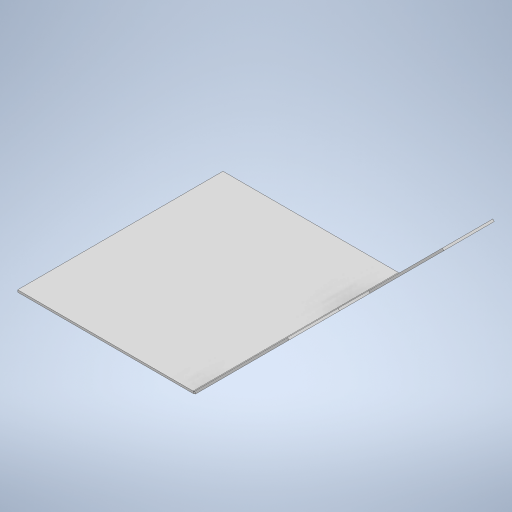
# Autodesk Inventor part: LzC-FrontPLateRS3
Saved by Autodesk Inventor 2024.3 (Build 283343000, 343)
## iProperties
Created: 2025-06-17
Part Number: LzC-FrontPLateRS3
Material: Generic
Document SubType Name: Sheet Metal
Designer: ajclo
Density: 1 g/cm^3
Sheet Metal Rule: Default_mm
Appearance: Default
Flat Pattern Width: 19.7 cm
Flat Pattern Length: 29.6736 cm
Flat Pattern Area: 584.57 cm^2
Sheet Metal Width: 197,000 mm
Sheet Metal Length: 296,736 mm
Sheet Metal Area: 58457,039 mm^2
Author: ajclo
Autodesk Inventor part; units mm, degrees
ref_plane "YZ Plane" through (0, 0, 0) normal (1, 0, 0) x (0, 1, 0)
ref_plane "XZ Plane" through (0, 0, 0) normal (0, 1, 0) x (-1, 0, 0)
ref_plane "XY Plane" through (0, 0, 0) normal (0, 0, 1) x (1, 0, 0)
sketch "Sketch1" plane through (0, 0, 0) normal (0, 1, 0) x (-1, 0, 0)
  line L0 (0, 0) -> (169.946, 0)
  line L1 (169.946, 0) -> (169.946, -197)
  line L2 (169.946, -197) -> (0, -197)
  line L3 (0, -197) -> (0, 0)
  dimension "d0" = 197
  dimension "d1" = 169.946
  measures "d0" distance of L0.end L1.end
  measures "d1" distance of L1.end L2.end
extrude "Plate1" add sketch "Sketch1" along normal blind 2
sketch "Sketch2" plane through (-1.4142, 1.4142, -197) normal (0.7071068, -0.7071068, 0) x (0.7071068, 0.7071068, 0)
  line L0 (0, 197) -> (0, 0)
  line L1 (0, 0) -> (127.842, 0)
  line L2 (127.842, 0) -> (127.842, 197)
  line L3 (127.842, 197) -> (0, 197)
  constraints: 6 end point, 1 horizontal, 1 perpendicular, 1 vertical
edge flange "Flange1" height 127.842 angle 45 thickness 2 bend radius 2 thickness toward (0.7071068, -0.7071068, 0) relief straight relief width 2 relief depth 1 edges at (0, 2, -98.5) wall of the first edge with corners at (-1.4142, 1.4142, 0) (-1.4142, 1.4142, -197) (88.9837, 91.8122, -197) (88.9837, 91.8122, 0)
bend "Bend1"
corner "Corner1"
sketch "Sketch3" plane through (90.3979, 90.3979, 0) normal (0.7071068, -0.7071068, 0) x (-0.7071068, -0.7071068, 0)
  line L0 (0, 48.5) -> (100, 48.5)
  line L1 (100, 48.5) -> (100, 148.5)
  line L2 (100, 148.5) -> (0, 148.5)
  line L3 (0, 148.5) -> (0, 48.5)
  line L4 (0, 197) -> (126.1851, 197) projected
  line L5 (0, 0) -> (0, 197) projected
  point P0 (127.842, 0)
  point P1 (63.0926, 197)
  dimension "d13" = 100
  dimension "d14" = 100
  dimension "d15" = 48.5
  constraints: 8 end point, 2 parallel, 1 collinear, 1 horizontal, 1 midpoint, 1 perpendicular
  measures "d13" distance of L2.end L0.start
  measures "d14" distance of L1.end L2.end
  measures "d15" distance from line of point (63.093, 197) L2
extrude "Cut1" cut sketch "Sketch3" against normal blind 2
equation "\"d14\" = d13"
equation "\"d16\" = Thickness"
equation "\"d2\" = Thickness"
equation "\"d3\" = BendReliefWidth"
equation "\"d4\" = BendReliefDepth"
equation "\"d5\" = MinimumRemnant"
equation "\"d6\" = TransitionRadius"
equation "\"d9\" = BendRadius"
equation "\"d10\" = CornerReliefSize"
equation "\"d11\" = GapSize"
equation "\"d12\" = JacobiRadiusSize"
equation "\"BendRadius\" = Thickness"
equation "\"BendReliefWidth\" = Thickness"
equation "\"BendReliefDepth\" = 0.5 * Thickness"
equation "\"CornerReliefSize\" = 4 * Thickness"
equation "\"MinimumRemnant\" = 2 * Thickness"
equation "\"TransitionRadius\" = BendRadius"
equation "\"JacobiRadiusSize\" = BendRadius"
equation "\"GapSize\" = Thickness"
equation "\"Thickness\" = 2"
body "Solid1"
